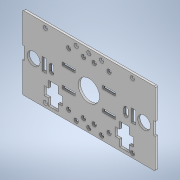
# Autodesk Inventor part: Зад
Saved by Autodesk Inventor 2021 (Build 250183000, 183)
## iProperties
Created: 2022-07-08
Part Number: Зад
Material: Типовые
Document SubType Name: Modeling
Designer: zvi20
Density: 1 g/cm^3
Appearance: По умолчанию
Author: zvi20
Autodesk Inventor part; units mm, degrees
ref_plane "YZ Plane" through (0, 0, 0) normal (1, 0, 0) x (0, 1, 0)
ref_plane "XZ Plane" through (0, 0, 0) normal (0, 1, 0) x (-1, 0, 0)
ref_plane "XY Plane" through (0, 0, 0) normal (0, 0, 1) x (1, 0, 0)
sketch "Эскиз1" plane through (0, 0, 0) normal (0, 0, 1) x (1, 0, 0)
  line L0 (15.9926, -16.8371) -> (138.9926, -16.8371)
  line L1 (139.9926, -17.8371) -> (139.9926, -45.3371)
  line L2 (139.9926, -45.3371) -> (138.4926, -45.3371)
  line L3 (138.4926, -45.3371) -> (138.4926, -57.3371)
  line L4 (138.4926, -57.3371) -> (139.9926, -57.3371)
  line L5 (139.9926, -57.3371) -> (139.9926, -84.8371)
  line L6 (138.9926, -85.8371) -> (15.9926, -85.8371)
  line L7 (14.9926, -84.8371) -> (14.9926, -57.3371)
  line L8 (14.9926, -57.3371) -> (16.4926, -57.3371)
  line L9 (16.4926, -57.3371) -> (16.4926, -45.3371)
  line L10 (16.4926, -45.3371) -> (14.9926, -45.3371)
  line L11 (14.9926, -45.3371) -> (14.9926, -17.8371)
  circle A0 centre (25.4926, -51.3371) radius 6
  circle A1 centre (129.4926, -51.3371) radius 6
  line L12 (33.4926, -57.3371) -> (33.4926, -45.3371)
  line L13 (33.4926, -45.3371) -> (37.4926, -45.3371)
  line L14 (37.4926, -45.3371) -> (37.4926, -57.3371)
  line L15 (37.4926, -57.3371) -> (33.4926, -57.3371)
  arc A2 (44.4926, -48.8371) -> (40.4926, -48.8371) centre (42.4926, -48.8371) ccw
  arc A3 (40.4926, -53.8371) -> (44.4926, -53.8371) centre (42.4926, -53.8371) ccw
  line L16 (44.4926, -53.8371) -> (44.4926, -48.8371)
  line L17 (40.4926, -53.8371) -> (40.4926, -48.8371)
  circle A4 centre (77.4926, -51.3371) radius 10
  line L18 (102.4926, -43.3371) -> (102.4926, -40.3371)
  line L19 (102.4926, -40.3371) -> (90.4926, -40.3371)
  line L20 (90.4926, -40.3371) -> (90.4926, -43.3371)
  line L21 (90.4926, -43.3371) -> (102.4926, -43.3371)
  circle A5 centre (77.4926, -20.8371) radius 2
  circle A6 centre (65.4926, -20.8371) radius 2
  circle A7 centre (89.4926, -20.8371) radius 2
  circle A8 centre (82.4926, -26.3371) radius 2
  circle A9 centre (118.4926, -20.8371) radius 2
  line L22 (106.4926, -61.8371) -> (106.4926, -68.3371)
  line L23 (106.4926, -68.3371) -> (102.4926, -68.3371)
  line L24 (102.4926, -68.3371) -> (102.4926, -76.3371)
  line L25 (102.4926, -76.3371) -> (106.4926, -76.3371)
  line L26 (115.4926, -61.8371) -> (106.4926, -61.8371)
  line L27 (115.4926, -68.3371) -> (115.4926, -61.8371)
  line L28 (106.4926, -76.3371) -> (106.4926, -82.8371)
  line L29 (106.4926, -82.8371) -> (115.4926, -82.8371)
  line L30 (115.4926, -82.8371) -> (115.4926, -76.3371)
  line L31 (115.4926, -76.3371) -> (119.4926, -76.3371)
  line L32 (119.4926, -68.3371) -> (115.4926, -68.3371)
  line L33 (119.4926, -76.3371) -> (119.4926, -68.3371)
  arc A10 (15.9926, -16.8371) -> (14.9926, -17.8371) centre (15.9926, -17.8371) ccw
  arc A11 (14.9926, -84.8371) -> (15.9926, -85.8371) centre (15.9926, -84.8371) ccw
  arc A12 (138.9926, -85.8371) -> (139.9926, -84.8371) centre (138.9926, -84.8371) ccw
  arc A13 (139.9926, -17.8371) -> (138.9926, -16.8371) centre (138.9926, -17.8371) ccw
  circle A14 centre (96.4926, -26.3371) radius 2
  circle A15 centre (58.4926, -26.3371) radius 2
  circle A16 centre (72.4926, -26.3371) radius 2
  circle A17 centre (36.4926, -20.8371) radius 2
  line L34 (102.4926, -59.3371) -> (102.4926, -62.3371)
  line L35 (102.4926, -62.3371) -> (90.4926, -62.3371)
  line L36 (90.4926, -62.3371) -> (90.4926, -59.3371)
  line L37 (90.4926, -59.3371) -> (102.4926, -59.3371)
  line L38 (52.4926, -43.3371) -> (52.4926, -40.3371)
  line L39 (52.4926, -40.3371) -> (64.4926, -40.3371)
  line L40 (64.4926, -40.3371) -> (64.4926, -43.3371)
  line L41 (64.4926, -43.3371) -> (52.4926, -43.3371)
  line L42 (52.4926, -59.3371) -> (52.4926, -62.3371)
  line L43 (64.4926, -59.3371) -> (52.4926, -59.3371)
  line L44 (64.4926, -62.3371) -> (64.4926, -59.3371)
  line L45 (52.4926, -62.3371) -> (64.4926, -62.3371)
  line L46 (121.4926, -57.3371) -> (121.4926, -45.3371)
  line L47 (121.4926, -45.3371) -> (117.4926, -45.3371)
  line L48 (117.4926, -45.3371) -> (117.4926, -57.3371)
  line L49 (117.4926, -57.3371) -> (121.4926, -57.3371)
  arc A18 (114.4926, -48.8371) -> (110.4926, -48.8371) centre (112.4926, -48.8371) ccw
  arc A19 (110.4926, -53.8371) -> (114.4926, -53.8371) centre (112.4926, -53.8371) ccw
  line L50 (110.4926, -53.8371) -> (110.4926, -48.8371)
  line L51 (114.4926, -53.8371) -> (114.4926, -48.8371)
  line L52 (82.4926, -26.3371) -> (82.4926, -26.3371)
  circle A20 centre (77.4926, -81.8371) radius 2
  circle A21 centre (65.4926, -81.8371) radius 2
  circle A22 centre (89.4926, -81.8371) radius 2
  circle A23 centre (82.4926, -76.3371) radius 2
  circle A24 centre (118.4926, -81.8371) radius 2
  circle A25 centre (96.4926, -76.3371) radius 2
  circle A26 centre (58.4926, -76.3371) radius 2
  circle A27 centre (72.4926, -76.3371) radius 2
  circle A28 centre (36.4926, -81.8371) radius 2
  line L53 (39.4926, -61.8371) -> (48.4926, -61.8371)
  line L54 (39.4926, -68.3371) -> (39.4926, -61.8371)
  line L55 (48.4926, -61.8371) -> (48.4926, -68.3371)
  line L56 (48.4926, -68.3371) -> (52.4926, -68.3371)
  line L57 (52.4926, -68.3371) -> (52.4926, -76.3371)
  line L58 (52.4926, -76.3371) -> (48.4926, -76.3371)
  line L59 (48.4926, -82.8371) -> (39.4926, -82.8371)
  line L60 (48.4926, -76.3371) -> (48.4926, -82.8371)
  line L61 (39.4926, -82.8371) -> (39.4926, -76.3371)
  line L62 (39.4926, -76.3371) -> (35.4926, -76.3371)
  line L63 (35.4926, -68.3371) -> (39.4926, -68.3371)
  line L64 (35.4926, -76.3371) -> (35.4926, -68.3371)
  point P0 (0, 0)
  point P1 (14.9926, -16.8371)
  point P2 (139.9926, -16.8371)
  point P3 (139.9926, -85.8371)
  point P4 (34.4926, -62.3371)
  point P5 (51.4926, -81.3371)
  point P6 (119.9926, -62.3371)
  point P7 (102.9926, -81.3371)
  point P8 (118.4926, -81.3371)
  constraints: 130 end point, 29 centre point, 26 point on line, 16 point on circle, 14 perpendicular, 9 tangent, 3 equal radius, 2 horizontal, 2 vertical
extrude "Выдавливание3" add sketch "Эскиз1" along normal blind 2
